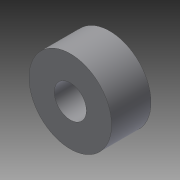
# Autodesk Inventor part: Joint_Magnet
Saved by Autodesk Inventor 2014 (Build 180170000, 170)
## iProperties
Created: 2014-08-27
Part Number: Joint_Magnet
Material: Generic
Document SubType Name: Modeling
Designer: ThatOtherGuy
Density: 1 g/cm^3
Appearance: Default
Author: ThatOtherGuy
Autodesk Inventor part; units mm, degrees
ref_plane "YZ Plane" through (0, 0, 0) normal (1, 0, 0) x (0, 1, 0)
ref_plane "XZ Plane" through (0, 0, 0) normal (0, 1, 0) x (-1, 0, 0)
ref_plane "XY Plane" through (0, 0, 0) normal (0, 0, 1) x (1, 0, 0)
sketch "Sketch1" plane through (0, 0, 0) normal (0, 0, 1) x (1, 0, 0)
  line L0 (1.9, 0) -> (1.9, 3)
  line L1 (4.4153, 4.65) -> (4.75, 4.65)
  line L2 (4.75, 4.65) -> (4.75, 0)
  line L3 (4.75, 0) -> (1.9, 0)
  line L4 (0, 0) -> (0, 3)
  arc A0 (1.9, 3) -> (4.4153, 4.65) centre (0, 8.6385) ccw
  dimension "d0" = 4.65
  dimension "d2" = 4.75
  dimension "d10" = 5.95
  dimension "d11" = 3
  dimension "d12" = 1.9
  constraints: 10 end point, 3 parallel, 2 perpendicular, 2 point on circle, 1 centre point, 1 horizontal alignment, 1 vertical, 1 vertical alignment
  measures "d0" distance of L1.end L2.end
  measures "d2" distance from line of L4.start L2
  measures "d10" radius of A0
  measures "d11" distance of L0.start L0.end
  measures "d12" distance between parallel lines of L4 L0
revolve "Revolution1" add sketch "Sketch1" angle 360 about axis through (0, 0, 0) along (0, 1, 0)
equation "\"d2\" = 0.5 * MAGDIA"
equation "\"THICKA\" = 3.175"
equation "\"THICKB\" = 6.731"
equation "\"THICKC\" = 12.7"
equation "\"MAGDIA\" = 9.5"
equation "\"BALLDIA\" = 12"
equation "\"THICKPLY\" = 5"
body "Solid1"
